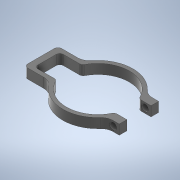
# Autodesk Inventor part: vibrator holder
Saved by Autodesk Inventor 2020.2 (Build 242310000, 310)
## iProperties
Created: 2020-10-29
Part Number: vibrator holder
Material: Generic
Document SubType Name: Modeling
Designer: JK
Density: 1 g/cm^3
Appearance: Smooth - Black
Author: JK
Autodesk Inventor part; units mm, degrees
ref_plane "YZ Plane" through (0, 0, 0) normal (1, 0, 0) x (0, 1, 0)
ref_plane "XZ Plane" through (0, 0, 0) normal (0, 1, 0) x (-1, 0, 0)
ref_plane "XY Plane" through (0, 0, 0) normal (0, 0, 1) x (1, 0, 0)
sketch "Sketch1" plane through (0, 0, 0) normal (0, 1, 0) x (-1, 0, 0)
  circle A0 centre (0, 0) radius 26
  circle A1 centre (0, 0) radius 29
  line L0 (-24, 27.6963) -> (-41.2964, 27.6963)
  line L1 (-41.2964, 27.6963) -> (-41.2964, -30.0075)
  line L2 (-41.2964, -30.0075) -> (-24, -30.0075)
  line L3 (-24, -30.0075) -> (-24, 27.6963)
  point P0 (-24, 16.2788)
  point P1 (-24, 10)
  point P2 (-24, -10)
  point P3 (-24, -16.2788)
  dimension "d0" = 52
  dimension "d1" = 24
  dimension "d7" = 3
  constraints: 8 end point, 2 centre point, 2 coincident, 2 parallel, 1 horizontal, 1 perpendicular
  measures "d0" diameter of A0
  measures "d1" distance from line of point (0, 0) L3
  measures "d7" radial gap between concentric circles of A0 A1
extrude "Extrusion1" add sketch "Sketch1" along normal blind 8 contours A0 L3 A1 picked at (-1.374, -26.8299)
sketch "Sketch3" plane through (0, 8, 0) normal (0, 1, 0) x (1, 0, 0)
  line L0 (-42, -10.5) -> (-26, -10.5)
  line L1 (-26, -10.5) -> (-26, 10.5)
  line L2 (-26, 10.5) -> (-42, 10.5)
  line L3 (-42, 10.5) -> (-42, -10.5)
  line L4 (-42, -10.5) -> (-26, 10.5) construction
  line L5 (-26, -10.5) -> (-42, 10.5) construction
  arc A0 (24, 10) -> (24, -10) centre (0, 0) ccw projected
  line L6 (-42, 10.5) -> (-12.6502, 10.5)
  line L7 (-12.6502, 10.5) -> (-12.6502, -10.5)
  line L8 (-12.6502, -10.5) -> (-42, -10.5)
  line L9 (-42, -10.5) -> (-42, 10.5)
  point P0 (-34, 0)
  dimension "d16" = 0
  dimension "d17" = 10.5
  dimension "d18" = 16
  constraints: 20 end point, 4 parallel, 2 horizontal, 2 midpoint, 2 perpendicular, 1 tangent
  measures "d16" vertical distance of point (0, 0) point (-34, 0)
  measures "d17" distance from line of point (0, 0) L0
  measures "d18" distance between parallel lines of L1 L3
extrude "Extrusion3" cut sketch "Sketch3" against normal blind 10
sketch "Sketch4" plane through (0, 8, 0) normal (0, 1, 0) x (1, 0, 0)
  circle A0 centre (0, 0) radius 26
  line L0 (-27.0324, 10.5) -> (-23.7855, 10.5) projected
  line L1 (-55.2626, -10.5) -> (-23.7855, -10.5)
  line L2 (-23.7855, -10.5) -> (-23.7855, 10.5)
  line L3 (-23.7855, 10.5) -> (-55.2626, 10.5)
  line L4 (-55.2626, 10.5) -> (-55.2626, -10.5)
  line L5 (-55.2626, -10.5) -> (-23.7855, 10.5) construction
  line L6 (-23.7855, -10.5) -> (-55.2626, 10.5) construction
  arc A1 (-27.0324, -10.5) -> (24, -16.2788) centre (0, 0) ccw projected
  line L7 (-43.0324, 10.5) -> (-27.0324, 10.5)
  line L8 (-27.0324, 10.5) -> (-27.0324, -10.5)
  line L9 (-27.0324, -10.5) -> (-43.0324, -10.5)
  line L10 (-43.0324, -10.5) -> (-43.0324, 10.5)
  line L11 (-43.0324, 10.5) -> (-27.0324, -10.5) construction
  line L12 (-27.0324, 10.5) -> (-43.0324, -10.5) construction
  line L13 (-47.0324, 14) -> (-25.3969, 14)
  line L14 (-25.3969, 14) -> (-25.3969, -14)
  line L15 (-25.3969, -14) -> (-47.0324, -14)
  line L16 (-47.0324, -14) -> (-47.0324, 14)
  line L17 (-27.0324, -10.5) -> (-23.7855, -10.5) projected
  line L18 (-26, -10.5) -> (-26, 10.5)
  line L19 (-43.0324, 10.5) -> (-42.0324, 10.5)
  line L20 (-42.0324, 10.5) -> (-42.0324, -10.5)
  line L21 (-42.0324, -10.5) -> (-43.0324, -10.5)
  line L22 (-43.0324, -10.5) -> (-43.0324, 10.5)
  point P0 (-39.524, 0)
  point P1 (-35.0324, 0)
  point P2 (-25.3969, -10.5)
  point P3 (-43.0324, -10.5)
  point P4 (-43.0324, 10.5)
  point P5 (-25.3969, 10.5)
  dimension "d21" = 16
  dimension "d22" = 14
  dimension "d23" = 14
  dimension "d24" = 4
  dimension "d27" = 21
  dimension "d37" = 1
  constraints: 43 end point, 8 parallel, 5 perpendicular, 4 horizontal, 4 midpoint, 3 point on line, 1 coincident, 1 point on circle, 3 other
  measures "d21" distance between parallel lines of L10 L8
  measures "d22" distance from line of L13 point (0, 0)
  measures "d23" distance from line of L15 point (0, 0)
  measures "d24" distance between parallel lines of L16 L10
  measures "d27" distance between parallel lines of L7 L1
  measures "d37" distance between parallel lines of L20 L22
extrude "Extrusion4" add sketch "Sketch4" against normal up to surface (8 mm away) contours L0 L3 L16 L13 L14 | L14 A1 L1 | L15 L16 L1 A1 | L20 L1 L10 L3 | L3 L10 L1 L16
sketch "Sketch5" plane through (0, 8, 0) normal (0, 1, 0) x (1, 0, 0)
  line L0 (24, 16.2788) -> (34, 16.2788)
  line L1 (34, 16.2788) -> (34, 10)
  line L2 (34, 10) -> (24, 10)
  line L3 (24, 10) -> (24, 16.2788)
  arc A0 (-23.7855, -10.5) -> (24, -10) centre (0, 0) ccw projected
  line L4 (24, -10) -> (34, -10)
  line L5 (34, -10) -> (34, -16.2788)
  line L6 (34, -16.2788) -> (24, -16.2788)
  line L7 (24, -16.2788) -> (24, -10)
  dimension "d30" = 10
  constraints: 16 end point, 4 parallel, 2 coincident, 2 horizontal, 2 perpendicular, 1 collinear
  measures "d30" distance from line of L1 point (24, 10)
extrude "Extrusion5" add sketch "Sketch5" against normal up to surface (8 mm away)
sketch "Sketch6" plane through (24, 8, 16.2788) normal (0, 0, 1) x (1, 0, 0)
  circle A0 centre (5.0293, -4) radius 2.75
  line L0 (10, -8) -> (0, -8) projected
  point P0 (-24, -8)
  dimension "d31" = 4
  dimension "d32" = 5.5
  constraints: 1 centre point
  measures "d31" distance from line of A0.centre L0
  measures "d32" diameter of A0
extrude "Extrusion6" cut sketch "Sketch6" against normal through all
fillet "Fillet1" radius 10 4 edges at (-25.3969, 4, 14) (24, 4, 16.2788) (24, 4, -16.2788) (-25.3969, 4, -14)
fillet "Fillet2" radius 3 8 edges at (-47.0324, 4, -14) (-47.0324, 4, 14) (-23.7855, 4, -10.5) (-23.7855, 4, 10.5) (24, 4, -10) (24, 4, 10) (-42.0324, 4, -10.5) (-42.0324, 4, 10.5)
sketch "Sketch2" plane through (0, 8, 0) normal (0, 1, 0) x (1, 0, 0)
  line L0 (-43.8438, 10.5) -> (-27.8438, 10.5)
  line L1 (-27.8438, 10.5) -> (-27.8438, -10.5)
  line L2 (-27.8438, -10.5) -> (-43.8438, -10.5)
  line L3 (-43.8438, -10.5) -> (-43.8438, 10.5)
  line L4 (-43.8438, 10.5) -> (-27.8438, -10.5) construction
  line L5 (-27.8438, 10.5) -> (-43.8438, -10.5) construction
  line L6 (-46.8438, 13.5) -> (-24.8438, 13.5)
  line L7 (-24.8438, 13.5) -> (-24.8438, -13.5)
  line L8 (-24.8438, -13.5) -> (-46.8438, -13.5)
  line L9 (-46.8438, -13.5) -> (-46.8438, 13.5)
  line L10 (-46.8438, 13.5) -> (-24.8438, -13.5) construction
  line L11 (-24.8438, 13.5) -> (-46.8438, -13.5) construction
  arc A0 (24, 16.2788) -> (24, -16.2788) centre (0, 0) ccw projected
  line L12 (-17.6252, 23.0294) -> (-24.8438, 23.0294)
  line L13 (-24.8438, 23.0294) -> (-24.8438, -13.5)
  line L14 (-24.8438, -13.5) -> (-17.6252, -13.5)
  line L15 (-17.6252, -13.5) -> (-17.6252, 23.0294)
  arc A1 (24, 10) -> (24, -10) centre (0, 0) ccw projected
  point P0 (-35.8438, 0)
  point P1 (-35.8438, 0)
  point P2 (-10.332, -13.5)
  dimension "d10" = 3
  dimension "d11" = 3
  dimension "d12" = 21
  dimension "d13" = 16
  constraints: 32 end point, 6 parallel, 5 midpoint, 3 horizontal, 3 perpendicular, 1 point on circle
  measures "d10" distance between parallel lines of L8 L2
  measures "d11" distance between parallel lines of L7 L1
  measures "d12" distance between parallel lines of L2 L0
  measures "d13" distance between parallel lines of L1 L3
body "Solid1"
